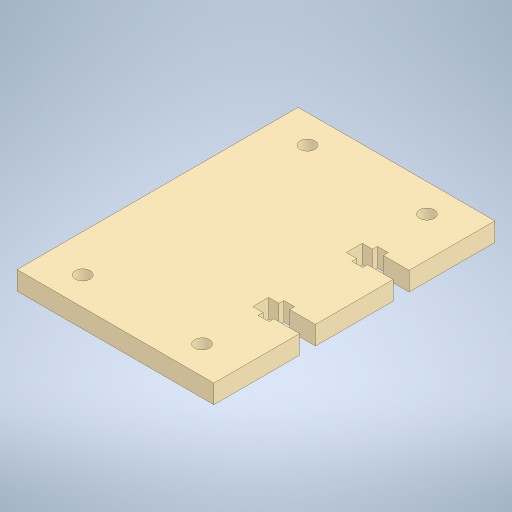
# Autodesk Inventor part: каретки_потолок
Saved by Autodesk Inventor 2023.1 (Build 271208000, 208)
## iProperties
Created: 2026-02-03
Part Number: каретки_потолок
Material: Типовые
Document SubType Name: Modeling
Designer: DELL
Density: 1 g/cm^3
Appearance: Бежевый
Author: DELL
Autodesk Inventor part; units mm, degrees
ref_plane "YZ Plane" through (0, 0, 0) normal (1, 0, 0) x (0, 1, 0)
ref_plane "XZ Plane" through (0, 0, 0) normal (0, 1, 0) x (-1, 0, 0)
ref_plane "XY Plane" through (0, 0, 0) normal (0, 0, 1) x (1, 0, 0)
sketch "Эскиз1" plane through (0, 0, 0) normal (0, 1, 0) x (-1, 0, 0)
  line L0 (21, 30) -> (-21, 30)
  line L1 (-21, 30) -> (-21, -30)
  line L2 (-21, -30) -> (21, -30)
  line L3 (21, -30) -> (21, 30)
  line L4 (21, 30) -> (-21, -30) construction
  line L5 (-21, 30) -> (21, -30) construction
  point P0 (0, 0)
  dimension "d0" = 42
  dimension "d1" = 60
  constraints: 12 end point, 2 midpoint, 2 parallel, 1 horizontal, 1 perpendicular
  measures "d0" distance of L2.end L1.end
  measures "d1" distance of L1.end L0.end
extrude "Выдавливание1" add sketch "Эскиз1" along normal blind 4
sketch "Эскиз4" plane through (0, 4, 0) normal (0, 1, 0) x (1, 0, 0)
  circle A0 centre (-13, -24) radius 1.6
  circle A1 centre (12.5, -24) radius 1.6
  circle A2 centre (12.5, 24) radius 1.6
  circle A3 centre (-13, 24) radius 1.6
  line L0 (-21, 30) -> (-21, -30) projected
  line L1 (-21, -30) -> (21, -30) projected
  line L2 (21, -30) -> (21, 30) projected
  line L3 (21, 30) -> (-21, 30) projected
  point P0 (0, 0)
  dimension "d28" = 3.2
  dimension "d29" = 3.2
  dimension "d31" = 3.2
  dimension "d32" = 8
  dimension "d33" = 6
  dimension "d34" = 6
  dimension "d36" = 6
  dimension "d37" = 6
  dimension "d38" = 8
  dimension "d56" = 25.5
  dimension "d57" = 3.2
  dimension "d58" = 25.5
  constraints: 4 centre point
  measures "d28" diameter of A0
  measures "d29" diameter of A1
  measures "d31" diameter of A3
  measures "d32" distance from line of L0 A0.centre
  measures "d33" distance from line of L1 A0.centre
  measures "d34" distance from line of L1 A1.centre
  measures "d36" distance from line of L3 A2.centre
  measures "d37" distance from line of L3 A3.centre
  measures "d38" distance from line of L0 A3.centre
  measures "d56" distance of A1.centre A0.centre
  measures "d57" diameter of A2
  measures "d58" distance of A3.centre A2.centre
extrude "Выдавливание3" cut sketch "Эскиз4" against normal blind 10 contours A0 | A1 | A2 | A3
sketch "Эскиз5" plane through (0, 4, 0) normal (0, 1, 0) x (1, 0, 0)
  line L0 (21, -30) -> (21, 30) projected
  line L1 (21, -8.3) -> (11, -8.3)
  line L2 (11, -8.3) -> (11, -11.7)
  line L3 (11, -11.7) -> (21, -11.7)
  line L4 (21, -11.7) -> (21, -8.3)
  line L5 (21, 8.3) -> (11, 8.3)
  line L6 (11, 8.3) -> (11, 11.7)
  line L7 (11, 11.7) -> (21, 11.7)
  line L8 (21, 11.7) -> (21, 8.3)
  line L9 (0, 0) -> (21, 0) construction
  line L10 (15.5, -7.25) -> (13.2, -7.25)
  line L11 (13.2, -7.25) -> (13.2, -12.75)
  line L12 (13.2, -12.75) -> (15.5, -12.75)
  line L13 (15.5, -12.75) -> (15.5, -7.25)
  line L14 (15.5, -7.25) -> (13.2, -12.75) construction
  line L15 (13.2, -7.25) -> (15.5, -12.75) construction
  line L16 (13.2, 7.25) -> (15.5, 7.25)
  line L17 (15.5, 7.25) -> (15.5, 12.75)
  line L18 (15.5, 12.75) -> (13.2, 12.75)
  line L19 (13.2, 12.75) -> (13.2, 7.25)
  line L20 (13.2, 7.25) -> (15.5, 12.75) construction
  line L21 (15.5, 7.25) -> (13.2, 12.75) construction
  point P0 (21, -10)
  point P1 (21, 10)
  point P2 (14.35, -10)
  point P3 (14.35, 10)
  point P4 (15.5, -10)
  point P5 (15.5, -11.7)
  point P6 (21, -11.7)
  point P7 (15.5, -8.3)
  point P8 (13.2, -8.3)
  point P9 (13.2, -11.7)
  point P10 (13.2, 8.3)
  point P11 (15.5, 8.3)
  point P12 (21, 8.3)
  point P13 (21, 11.7)
  point P14 (15.5, 11.7)
  point P15 (13.2, 11.7)
  dimension "d42" = 10
  dimension "d43" = 3.4
  dimension "d44" = 10
  dimension "d45" = 3.4
  dimension "d46" = 10
  dimension "d47" = 10
  dimension "d48" = 2.3
  dimension "d49" = 5.5
  dimension "d50" = 2.3
  dimension "d51" = 5.5
  dimension "d52" = 5.5
  dimension "d53" = 5.5
  constraints: 42 end point, 8 midpoint, 8 parallel, 4 horizontal, 4 perpendicular, 2 point on line
  measures "d42" distance of L3.end L2.end
  measures "d43" distance of L2.end L1.end
  measures "d44" distance of L6.end L7.end
  measures "d45" distance of L5.end L6.end
  measures "d46" distance from line of point (21, -10) L9
  measures "d47" distance from line of point (21, 10) L9
  measures "d48" distance of L12.end L11.end
  measures "d49" distance of L11.end L10.end
  measures "d50" distance of L18.end L17.end
  measures "d51" distance of L17.end L16.end
  measures "d52" distance from line of L0 point (15.5, -10)
  measures "d53" distance between parallel lines of L8 L17
extrude "Выдавливание4" cut sketch "Эскиз5" against normal blind 4
